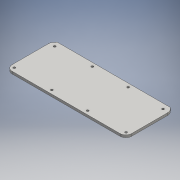
# Autodesk Inventor part: Housing cover
Saved by Autodesk Inventor 2016 (Build 200138000, 138)
## iProperties
Created: 2019-09-20
Part Number: Housing cover
Material: Generic
Document SubType Name: Modeling
Designer: jimmy
Density: 1 g/cm^3
Appearance: Default
Author: jimmy
Autodesk Inventor part; units mm, degrees
ref_plane "YZ Plane" through (0, 0, 0) normal (1, 0, 0) x (0, 1, 0)
ref_plane "XZ Plane" through (0, 0, 0) normal (0, 1, 0) x (-1, 0, 0)
ref_plane "XY Plane" through (0, 0, 0) normal (0, 0, 1) x (1, 0, 0)
sketch "Sketch1" plane through (0, 0, 0) normal (0, 0, 1) x (1, 0, 0)
  line L0 (30, 31.5) -> (34, 31.5)
  line L1 (34, 36) -> (34, 31.5)
  arc A0 (34, 36) -> (44, 46) centre (34, 46) ccw
  line L2 (44, 46) -> (106, 46)
  arc A1 (106, 46) -> (121, 31) centre (121, 46) ccw
  line L3 (121, 31) -> (121, -29.2696)
  arc A2 (104.9089, -46) -> (121, -29.2696) centre (15.3991, 56.1924) ccw
  line L4 (104.9089, -46) -> (44, -46)
  arc A3 (44, -46) -> (34, -36) centre (34, -46) ccw
  line L5 (34, -21.5) -> (34, -36)
  line L6 (34, -21.5) -> (30, -21.5)
  line L7 (30, -46) -> (30, -21.5)
  line L8 (30, -46) -> (-30, -46)
  line L9 (-30, -21.5) -> (-30, -46)
  line L10 (-30, -21.5) -> (-34, -21.5)
  line L11 (-34, -36) -> (-34, -21.5)
  arc A4 (-34, -36) -> (-44, -46) centre (-34, -46) ccw
  line L12 (-44, -46) -> (-104.9089, -46)
  arc A5 (-121, -29.2696) -> (-104.9089, -46) centre (-15.3991, 56.1924) ccw
  line L13 (-121, -29.2696) -> (-121, 31)
  arc A6 (-121, 31) -> (-106, 46) centre (-121, 46) ccw
  line L14 (-106, 46) -> (-44, 46)
  arc A7 (-44, 46) -> (-34, 36) centre (-34, 46) ccw
  line L15 (-34, 21.5) -> (-34, 36)
  line L16 (-34, 21.5) -> (-30, 21.5)
  line L17 (-30, 46) -> (-30, 21.5)
  line L18 (-30, 46) -> (30, 46)
  line L19 (30, 31.5) -> (30, 46)
  circle A8 centre (-113.5, 39.5) radius 2.25
  circle A9 centre (-117.0823, -41.3881) radius 2.25
  circle A10 centre (-37.5, 42.5) radius 2.25
  circle A11 centre (-37.5, -42.5) radius 2.25
  arc A12 (-125, -38) -> (-113, -50) centre (-113, -38) ccw
  line L20 (-113, -50) -> (113, -50)
  arc A13 (113, -50) -> (125, -38) centre (113, -38) ccw
  line L21 (125, -38) -> (125, 38)
  arc A14 (125, 38) -> (120.5425, 47.3333) centre (113, 38) ccw
  line L22 (120.5425, 47.3333) -> (118.6569, 50)
  line L23 (-118.6569, 50) -> (118.6569, 50)
  line L24 (-120.5425, 47.3333) -> (-118.6569, 50)
  arc A15 (-120.5425, 47.3333) -> (-125, 38) centre (-113, 38) ccw
  line L25 (-125, 38) -> (-125, -38)
  circle A16 centre (117.0823, -41.3881) radius 2.25
  circle A17 centre (37.5, 42.5) radius 2.25
  circle A18 centre (113.5, 39.5) radius 2.25
  circle A19 centre (37.5, -42.5) radius 2.25
  point P0 (0, 0)
  point P1 (0, 0)
  constraints: 52 end point, 24 point on circle, 20 centre point
extrude "Extrusion1" add sketch "Sketch1" along normal blind 5 contours L0 L1 A0 L2 A1 L3 A2 L4 A3 L5 L6 L7 L8 L9 L10 L11 A4 L12 A5 L13 A6 L14 A7 L15 L16 L17 L18 L19 | L25 A15 L24 L23 L22 A14 L21 A13 L20 A12
body "Solid1"
